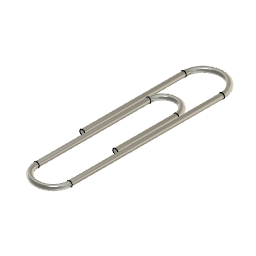
回形针 v1 (Autodesk Fusion 360 design; units mm, degrees)
Autodesk Fusion 360 part; units mm, degrees
sketch "草图1" plane through (0, 0, 0) normal (0, 0, 1) x (1, 0, 0) in component "paper clip"
  line L0 (0, 0) -> (0, 20)
  arc A0 (7.5, 20.0051) -> (0, 20) centre (3.75, 20) ccw
  line L1 (7.5, 20.0051) -> (7.5, -9.9949)
  arc A1 (1, -9.9949) -> (7.5, -9.9949) centre (4.25, -9.9949) ccw
  line L2 (1, -9.9949) -> (1, 12.0051)
  arc A2 (6.5, 12.0051) -> (1, 12.0051) centre (3.75, 12.0051) ccw
  line L3 (6.5, 12.0051) -> (6.5, 0.0051)
  dimension "d1" = 20
  dimension "d2" = 7.5
  dimension "d3" = 30
  dimension "d4" = 22
  dimension "d5" = 12
  constraint vertical L0
  constraint coincident L0.start origin
  constraint tangent L0 A0
  constraint vertical L1
  constraint tangent L1 A1
  constraint vertical L2
  constraint tangent L2 A2
  constraint parallel L1 L3
  measures "d1" distance of L0.start L0.end
  measures "d2" distance of L0.end A0.start
  measures "d3" distance of A0.start L1.end
  measures "d4" distance of A1.start L2.end
  measures "d5" distance of A2.start L3.end
sketch "草图2" plane through (0, 0, 0) normal (0, 1, 0) x (1, 0, 0) in component "paper clip"
  circle A0 centre (0, 0) radius 0.5
  dimension "d6" = 1
  constraint coincident A0.centre origin
  measures "d6" diameter of A0
sweep "扫掠1" add profiles "草图2" path "草图1" along L0 A0 L1 A1 L2 A2 L3 section 1 in component "paper clip"
component "paper clip" placed x (1, 0, 0) y (0, 1, 0) z (0, 0, 1) at (0, 0, 0)
